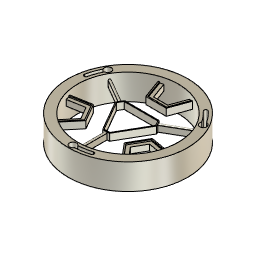
外壳1 v19 (Autodesk Fusion 360 design; units mm, degrees)
Autodesk Fusion 360 part; units mm, degrees
sketch "草图1" plane through (0, 0, 0) normal (0, 0, 1) x (1, 0, 0)
  circle A0 centre (0, 0) radius 43.1
  circle A1 centre (0, 0) radius 51.1
  circle A2 centre (0, 0) radius 44.72 construction
  line L0 (0.9412, -43.0897) -> (37.7874, 20.7297)
  line L1 (36.8462, 22.36) -> (-36.8462, 22.36)
  line L2 (-37.7874, 20.7297) -> (-0.9412, -43.0897)
  circle A3 centre (0, 0) radius 11.1 construction
  circle A4 centre (0, 0) radius 11.9 construction
  line L3 (-16.7613, 6.8314) -> (-2.4645, -17.9314)
  line L4 (2.4645, -17.9314) -> (16.7613, 6.8314)
  line L5 (14.2969, 11.1) -> (-14.2969, 11.1)
  line L6 (-17.6474, 6.7661) -> (-2.964, -18.6661)
  line L7 (2.964, -18.6661) -> (17.6474, 6.7661)
  line L8 (14.6833, 11.9) -> (-14.6833, 11.9)
  arc A5 (16.7613, 6.8314) -> (14.2969, 11.1) centre (0, 0) ccw
  arc A6 (17.6474, 6.7661) -> (14.6833, 11.9) centre (0, 0) ccw
  arc A7 (-14.2969, 11.1) -> (-16.7613, 6.8314) centre (0, 0) ccw
  arc A8 (-2.4645, -17.9314) -> (2.4645, -17.9314) centre (0, 0) ccw
  arc A9 (-14.6833, 11.9) -> (-17.6474, 6.7661) centre (0, 0) ccw
  arc A10 (-2.964, -18.6661) -> (2.964, -18.6661) centre (0, 0) ccw
  line L9 (0.9, -11.0635) -> (0.9, -11.8659)
  line L10 (0.9, -18.8786) -> (0.9, -43.1)
  line L11 (-0.9, -11.0635) -> (-0.9, -11.8659)
  line L12 (-0.9, -18.8786) -> (-0.9, -43.1)
  line L13 (0, -11.1) -> (0, -11.9)
  line L14 (16.7993, 8.6599) -> (37.7757, 20.7706)
  line L15 (15.8993, 10.2187) -> (36.8757, 22.3294)
  line L16 (-15.8993, 10.2187) -> (-36.8757, 22.3294)
  line L17 (-16.7993, 8.6599) -> (-37.7757, 20.7706)
  line L18 (0, 0) -> (0, -51.1) construction
  line L19 (0, 0) -> (-41.5692, 24) construction
  line L20 (0, 0) -> (48, 0) construction
  line L21 (0, 0) -> (43.1, 0) construction
  line L22 (0, 0) -> (43.1, 0) construction
  line L23 (-25.1627, -4.4369) -> (-16.4238, -19.5731)
  line L24 (-25.1627, -4.4369) -> (-42.4452, -7.4842)
  line L25 (-16.4238, -19.5731) -> (-27.7041, -33.0165)
  line L26 (-17.6399, -19.4667) -> (-28.4702, -32.3737)
  line L27 (-25.6787, -5.5433) -> (-17.6399, -19.4667)
  line L28 (-25.6787, -5.5433) -> (-42.2716, -8.469)
  line L29 (-21.1667, -19.1582) -> (-30.6917, -30.5096)
  line L30 (-27.1748, -8.7518) -> (-21.1667, -19.1582)
  line L31 (-27.1748, -8.7518) -> (-41.768, -11.325)
  line L32 (21.1667, -19.1582) -> (30.6917, -30.5096)
  line L33 (17.6399, -19.4667) -> (28.4702, -32.3737)
  line L34 (16.4238, -19.5731) -> (27.7041, -33.0165)
  line L35 (16.4238, -19.5731) -> (25.1627, -4.4369)
  line L36 (17.6399, -19.4667) -> (25.6787, -5.5433)
  line L37 (21.1667, -19.1582) -> (27.1748, -8.7518)
  line L38 (27.1748, -8.7518) -> (41.768, -11.325)
  line L39 (25.6787, -5.5433) -> (42.2716, -8.469)
  line L40 (25.1627, -4.4369) -> (42.4452, -7.4842)
  line L41 (6.0081, 27.91) -> (11.0763, 41.8346)
  line L42 (8.0387, 25.01) -> (13.8014, 40.8428)
  line L43 (8.7389, 24.01) -> (14.7411, 40.5008)
  line L44 (8.7389, 24.01) -> (-8.7389, 24.01)
  line L45 (8.0387, 25.01) -> (-8.0387, 25.01)
  line L46 (6.0081, 27.91) -> (-6.0081, 27.91)
  line L47 (-6.0081, 27.91) -> (-11.0763, 41.8346)
  line L48 (-8.0387, 25.01) -> (-13.8014, 40.8428)
  line L49 (-8.7389, 24.01) -> (-14.7411, 40.5008)
  circle A11 centre (0, 0) radius 47.1 construction
  arc A12 (2.6381, -48.5283) -> (14.7507, -46.3074) centre (0, 0) ccw
  arc A13 (2.5554, -45.5283) -> (13.8402, -43.4489) centre (0, 0) ccw
  arc A14 (45.6, 0) -> (-39.4908, 22.8) centre (0, 0) ccw
  arc A15 (2.5554, -45.5283) -> (2.6381, -48.5283) centre (0, -47.1) ccw
  arc A16 (14.7507, -46.3074) -> (13.8402, -43.4489) centre (14.2954, -44.8782) ccw
  arc A17 (38.151, 24.9772) -> (40.7077, 26.5489) centre (40.7898, 23.55) ccw
  arc A18 (38.151, 24.9772) -> (30.7078, 33.7104) centre (0, 0) ccw
  arc A19 (40.7077, 26.5489) -> (32.728, 35.9282) centre (0, 0) ccw
  arc A20 (32.728, 35.9282) -> (30.7078, 33.7104) centre (31.7179, 34.8193) ccw
  arc A21 (-40.7064, 20.5512) -> (-43.3459, 21.9795) centre (-40.7898, 23.55) ccw
  arc A22 (-40.7064, 20.5512) -> (-44.548, 9.7385) centre (0, 0) ccw
  arc A23 (-43.3459, 21.9795) -> (-47.4788, 10.3792) centre (0, 0) ccw
  arc A24 (-47.4788, 10.3792) -> (-44.548, 9.7385) centre (-46.0134, 10.0589) ccw
  circle A25 centre (0, -47.1) radius 1.3
  circle A26 centre (-40.7898, 23.55) radius 1.3
  circle A27 centre (40.7898, 23.55) radius 1.3
  dimension "d1" = 102.2
  dimension "d2" = 86.2
  dimension "d3" = 89.44
  dimension "d5" = 22.2
  dimension "d6" = 23.8
  dimension "d7" = 36.2
  dimension "d8" = 37.8
  dimension "d10" = 1.8
  dimension "d12" = 360
  dimension "d14" = 48
  dimension "d15" = 120
  dimension "d18" = 1.65
  dimension "d19" = 1
  dimension "d20" = -3.9
  dimension "d22" = 360
  dimension "d31" = 94.2
  dimension "d32" = 6
  dimension "d33" = 3
  dimension "d35" = 360
  dimension "d43" = 2.6
  dimension "d44" = 2.6
  dimension "d45" = 2.6
  constraint coincident A0.centre A1.centre
  constraint coincident A0 L1.start
  constraint coincident A0 L0.end
  constraint coincident A0 L1.end
  constraint coincident A0 L2.start
  constraint coincident A0 L2.end
  constraint coincident A0 L0.start
  constraint concentric A0 A3
  constraint concentric A4 A7
  constraint concentric A5 A7
  constraint concentric A6 A9
  constraint concentric A7 A8
  constraint concentric A9 A10
  constraint vertical L13
  constraint symmetric L12.end L10.end L13
  constraint coincident A3 L11.start
  constraint coincident A3 L9.start
  constraint coincident A3 L13.start
  constraint coincident A4 L9.end
  constraint collinear L9 L10
  constraint coincident A4 L11.end
  constraint collinear L11 L12
  constraint coincident A4 L13.end
  constraint coincident A10 L12.start
  constraint coincident A10 L10.start
  constraint coincident A1 L18.end
  constraint vertical L18
  constraint horizontal L20
  constraint parallel L16 L19
  constraint horizontal L21
  constraint horizontal L22
  constraint parallel L2 L23
  constraint concentric A6 A11
  constraint coincident L18 A15.centre
  constraint coincident A11 A15.centre
  constraint coincident A11 A16.centre
  constraint concentric A5 A12
  constraint tangent A13 A16
  constraint tangent A12 A16
  constraint coincident L19 A14.end
  constraint coincident L20 A14.start
  constraint concentric A13 A14
  constraint concentric A15 A25
  constraint concentric A21 A26
  constraint concentric A17 A27
  measures "d1" diameter of A1
  measures "d2" diameter of A0
  measures "d3" diameter of A2
  measures "d5" diameter of A3
  measures "d6" diameter of A4
  measures "d7" diameter of A7
  measures "d8" diameter of A9
  measures "d10" distance of L10 L12
  measures "d14" distance of A0.centre L19.end
  measures "d15" angle of L18 L19
  measures "d18" distance of L2 L23
  measures "d31" diameter of A11
  measures "d32" diameter of A15
  measures "d33" diameter of A16
  measures "d43" diameter of A25
  measures "d44" diameter of A26
  measures "d45" diameter of A27
extrude "拉伸1" add sketch "草图1" along normal blind 6 contours A0 L33 L34 L35 L36 L39 L40 | A0 L42 L43 L44 L45 L48 L49 | A0 L23 L24 L25 L26 L27 L28 | A1 | A12 A13 A15 A16 | A14 A17 A18 A19 A20 | A14 A17 | A21 A22 A23 A24 | A25 | A26 | A27
extrude "拉伸2" add sketch "草图1" along normal blind 5 contours A0 L32 L33 L36 L37 L38 L39 | A0 L41 L42 L45 L46 L47 L48 | A0 L26 L27 L28 L29 L30 L31
extrude "拉伸3" add sketch "草图1" along normal blind 5.9 contours A0 A6 L14 L15 | L6 L7 L8 A6 A9 A10 | A0 A10 L10 L12 | A0 A9 L16 L17
fillet "圆角1" radius 0.9 6 edges at (-26.3834, 16.2717, 5.9) (-27.2834, 14.7129, 5.9) (26.3834, 16.2717, 5.9) (27.2834, 14.7129, 5.9) (-0.9, -30.9846, 5.9) (0.9, -30.9846, 5.9)
extrude "拉伸4" cut sketch "草图1" along normal up to surface (6 mm away) contours A12 A13 A15 A16 | A14 A17 A18 A19 A20 | A14 A17 | A21 A22 A23 A24 | A25 | A26 | A27
extrude "拉伸5" add sketch "草图1" against normal blind 6.5 contours A1
extrude "拉伸8" add sketch "草图1" against normal up to surface (1.5 mm away) from surface at -5 contours A12 A13 A15 A16 | A14 A17 A18 A19 A20 | A14 A17 | A21 A22 A23 A24
extrude "拉伸9" add 1 faces at (48.0826, -4.6799, -6.5) along direction (0, 0, -1) blind 5.5
extrude "拉伸10" cut 3 faces at (3.9757, -47.396, -5) (39.0583, 27.1411, -5) (-43.034, 20.2549, -5) along direction (0, 0, -1) blind 5
sketch "草图3" plane through (0, 0, 6) normal (0, 0, 1) x (-1, 0, 0)
  arc A0 (-2.6381, 48.5283) -> (-14.7507, 46.3074) centre (0, 0) ccw
  arc A1 (-2.5554, 45.5283) -> (-2.6381, 48.5283) centre (0, 47.1) ccw
  arc A2 (-2.5554, 45.5283) -> (-13.8402, 43.4489) centre (0, 0) ccw
  arc A3 (-14.7507, 46.3074) -> (-13.8402, 43.4489) centre (-14.2954, 44.8782) ccw
  arc A4 (-40.7077, -26.5489) -> (-32.728, -35.9282) centre (0, 0) ccw
  arc A5 (-38.151, -24.9772) -> (-40.7077, -26.5489) centre (-40.7898, -23.55) ccw
  arc A6 (-38.151, -24.9772) -> (-30.7078, -33.7104) centre (0, 0) ccw
  arc A7 (-32.728, -35.9282) -> (-30.7078, -33.7104) centre (-31.7179, -34.8193) ccw
  arc A8 (43.3459, -21.9795) -> (47.4788, -10.3792) centre (0, 0) ccw
  arc A9 (40.7064, -20.5512) -> (43.3459, -21.9795) centre (40.7898, -23.55) ccw
  arc A10 (40.7064, -20.5512) -> (44.548, -9.7385) centre (0, 0) ccw
  arc A11 (47.4788, -10.3792) -> (44.548, -9.7385) centre (46.0134, -10.0589) ccw
  line L0 (-13.7974, -40.8319) -> (-8.0387, -25.01)
  line L1 (-8.0387, -25.01) -> (8.0387, -25.01)
  line L2 (8.0387, -25.01) -> (13.7974, -40.8319)
  arc A12 (-13.7974, -40.8319) -> (13.7974, -40.8319) centre (0, 0) ccw
  line L3 (25.6787, 5.5433) -> (17.6399, 19.4667)
  line L4 (17.6399, 19.4667) -> (28.4627, 32.3648)
  arc A13 (42.2601, 8.467) -> (28.4627, 32.3648) centre (0, 0) ccw
  line L5 (42.2601, 8.467) -> (25.6787, 5.5433)
  line L6 (8.7389, -24.01) -> (-8.7389, -24.01)
  line L7 (-8.7389, -24.01) -> (-14.7411, -40.5008)
  arc A14 (-42.4452, 7.4842) -> (-14.7411, -40.5008) centre (0, 0) ccw
  line L8 (-42.4452, 7.4842) -> (-25.1627, 4.4369)
  line L9 (-25.1627, 4.4369) -> (-16.4238, 19.5731)
  line L10 (-16.4238, 19.5731) -> (-27.7041, 33.0165)
  arc A15 (27.7041, 33.0165) -> (-27.7041, 33.0165) centre (0, 0) ccw
  line L11 (27.7041, 33.0165) -> (16.4238, 19.5731)
  line L12 (16.4238, 19.5731) -> (25.1627, 4.4369)
  line L13 (25.1627, 4.4369) -> (42.4452, 7.4842)
  arc A16 (14.7411, -40.5008) -> (42.4452, 7.4842) centre (0, 0) ccw
  line L14 (14.7411, -40.5008) -> (8.7389, -24.01)
  line L15 (-28.4627, 32.3648) -> (-17.6399, 19.4667)
  line L16 (-17.6399, 19.4667) -> (-25.6787, 5.5433)
  line L17 (-25.6787, 5.5433) -> (-42.2601, 8.467)
  arc A17 (-28.4627, 32.3648) -> (-42.2601, 8.467) centre (0, 0) ccw
  circle A18 centre (0, 0) radius 51.1
  circle A19 centre (0, 0) radius 43.1
  circle A20 centre (0, 0) radius 51.1
  constraint coincident A0.centre A2.centre
  constraint coincident L13.end A19
  constraint concentric A19 A20
extrude "拉伸12" add sketch "草图3" along normal blind 4
